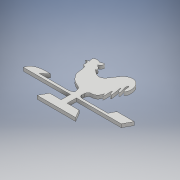
# Autodesk Inventor part: Part2
Saved by Autodesk Inventor 2017.1 (Build 211199000, 199)
## iProperties
Part Number: Part2
Material: 一般
Document SubType Name: Modeling
Designer: TomonoriSuzuki
Density: 1 g/cm^3
Appearance: 既定
Author: TomonoriSuzuki
Autodesk Inventor part; units mm, degrees
ref_plane "YZ Plane" through (0, 0, 0) normal (1, 0, 0) x (0, 1, 0)
ref_plane "XZ Plane" through (0, 0, 0) normal (0, 1, 0) x (-1, 0, 0)
ref_plane "XY Plane" through (0, 0, 0) normal (0, 0, 1) x (1, 0, 0)
sketch "スケッチ1" plane through (0, 0, 0) normal (0, 0, 1) x (1, 0, 0)
  line L0 (55.0072, -8.5794) -> (60.5037, 1.3591)
  line L1 (60.5037, 1.3591) -> (40.0223, 1.3591)
  line L2 (40.0223, 1.3591) -> (36.3075, -5.6978)
  line L3 (-44.8933, -5.4963) -> (-37.9032, 0.7038)
  line L4 (-37.9032, 0.7038) -> (-58.5109, 2.001) construction
  line L5 (-58.5109, 2.001) -> (-60.5622, -8.5794) construction
  spline S0 degree 2 poles (-37.9032, 0.7038) (-58.5109, 2.001) (-60.5622, -8.5794) knots 1 1 1 2 2 2
  line L6 (-15.656, 31.7874) -> (-2.1755, 18.5977) construction
  line L7 (-2.1755, 18.5977) -> (3.0159, 43.8698) construction
  line L8 (3.0159, 43.8698) -> (19.6839, 48.23) construction
  line L9 (19.6839, 48.23) -> (27.3182, 35.999) construction
  line L10 (27.3182, 35.999) -> (25.6769, 25.4506) construction
  line L11 (25.6769, 25.4506) -> (21.5058, 25.035) construction
  line L12 (21.5058, 25.035) -> (22.7873, 37.3838) construction
  line L13 (22.7873, 37.3838) -> (18.1485, 32.2406) construction
  line L14 (18.1485, 32.2406) -> (24.3226, 21.6179) construction
  line L15 (24.3226, 21.6179) -> (19.6839, 21.6179) construction
  line L16 (19.6839, 21.6179) -> (18.5132, 28.9494) construction
  line L17 (18.5132, 28.9494) -> (17.4163, 28.9494) construction
  line L18 (17.4163, 28.9494) -> (19.6839, 18.775) construction
  line L19 (19.6839, 18.775) -> (19.6839, 15.3221) construction
  spline S1 degree 4 poles (-15.656, 31.7874) (-2.1755, 18.5977) (3.0159, 43.8698) (19.6839, 48.23) (27.3182, 35.999) (25.6769, 25.4506) (21.5058, 25.035) (22.7873, 37.3838) (18.1485, 32.2406) (24.3226, 21.6179) (19.6839, 21.6179) (18.5132, 28.9494) (17.4163, 28.9494) (19.6839, 18.775) (19.6839, 15.3221) knots 1 1 1 1 1 2 3 4 5 6 7 8 9 10 11 12 12 12 12 12
  line L20 (19.6839, 15.3221) -> (18.1032, 13.7066) construction
  line L21 (18.1032, 13.7066) -> (16.92, 20.9253) construction
  line L22 (16.92, 20.9253) -> (15.2752, 20.6273) construction
  line L23 (15.2752, 20.6273) -> (16.92, 9.5318) construction
  line L24 (16.92, 9.5318) -> (15.3311, 6.9441) construction
  line L25 (15.3311, 6.9441) -> (14.2388, 16.1569) construction
  line L26 (14.2388, 16.1569) -> (14.2388, 5.6827) construction
  line L27 (14.2388, 5.6827) -> (6.7434, 3.9502) construction
  line L28 (6.7434, 3.9502) -> (3.9779, 5.6484) construction
  line L29 (3.9779, 5.6484) -> (2.3718, 1.2463) construction
  spline S2 degree 4 poles (19.6839, 15.3221) (18.1032, 13.7066) (16.92, 20.9253) (15.2752, 20.6273) (16.92, 9.5318) (15.3311, 6.9441) (14.2388, 16.1569) (14.2388, 5.6827) (6.7434, 3.9502) (3.9779, 5.6484) (2.3718, 1.2463) knots 1 1 1 1 1 2 3 4 5 6 7 8 8 8 8 8
  line L30 (2.3718, 1.2463) -> (2.0923, -2.1636) construction
  spline S3 degree 1 poles (2.3718, 1.2463) (2.0923, -2.1636) knots 1 1 2 2
  line L31 (-15.656, 31.7874) -> (-12.3988, 31.7874) construction
  line L32 (-12.3988, 31.7874) -> (-17.5466, 36.4877) construction
  line L33 (-17.5466, 36.4877) -> (-20.4147, 39.1064) construction
  line L34 (-20.4147, 39.1064) -> (-17.5466, 36.4877) construction
  line L35 (-17.5466, 36.4877) -> (-13.6458, 45.2036) construction
  line L36 (-13.6458, 45.2036) -> (-20.6141, 41.5266) construction
  line L37 (-20.6141, 41.5266) -> (-20.6142, 41.5266) construction
  line L38 (-20.6142, 41.5266) -> (-20.6136, 41.5266) construction
  line L39 (-20.6136, 41.5266) -> (-23.0367, 43.0844) construction
  line L40 (-23.0367, 43.0844) -> (-29.1871, 43.0844) construction
  line L41 (-29.1871, 43.0844) -> (-28.8447, 37.7285) construction
  line L42 (-28.8447, 37.7285) -> (-26.6696, 36.913) construction
  line L43 (-26.6696, 36.913) -> (-30.3539, 36.4706) construction
  line L44 (-30.3539, 36.4706) -> (-32.0674, 34.4706) construction
  line L45 (-32.0674, 34.4706) -> (-28.5043, 36.251) construction
  line L46 (-28.5043, 36.251) -> (-27.2474, 32.6902) construction
  line L47 (-27.2474, 32.6902) -> (-28.5043, 29.2574) construction
  line L48 (-28.5043, 29.2574) -> (-27.2474, 29.0008) construction
  line L49 (-27.2474, 29.0008) -> (-23.7709, 29.4706) construction
  line L50 (-23.7709, 29.4706) -> (-23.7709, 15.1294) construction
  line L51 (-23.7709, 15.1294) -> (-21.2036, 15.1294) construction
  line L52 (-21.2036, 15.1294) -> (-18.5996, 7.7294) construction
  line L53 (-18.5996, 7.7294) -> (-7.5699, 3.7053) construction
  line L54 (-7.5699, 3.7053) -> (-6.3253, 3.2512) construction
  line L55 (-6.3253, 3.2512) -> (-5.1075, -2.2999) construction
  spline S4 degree 4 poles (-15.656, 31.7874) (-12.3988, 31.7874) (-17.5466, 36.4877) (-20.4147, 39.1064) (-17.5466, 36.4877) (-13.6458, 45.2036) (-20.6141, 41.5266) (-20.6142, 41.5266) (-20.6136, 41.5266) (-23.0367, 43.0844) (-29.1871, 43.0844) (-28.8447, 37.7285) (-26.6696, 36.913) (-30.3539, 36.4706) (-32.0674, 34.4706) (-28.5043, 36.251) (-27.2474, 32.6902) (-28.5043, 29.2574) (-27.2474, 29.0008) (-23.7709, 29.4706) (-23.7709, 15.1294) (-21.2036, 15.1294) (-18.5996, 7.7294) (-7.5699, 3.7053) (-6.3253, 3.2512) (-5.1075, -2.2999) knots 1 1 1 1 1 2 3 4 5 6 7 8 9 10 11 12 13 14 15 16 17 18 19 20 21 22 23 23 23 23 23
  line L56 (-44.8933, -5.4963) -> (-13.2475, -5.4963)
  line L57 (36.3075, -5.6978) -> (6.9345, -5.6978)
  line L58 (6.9345, -5.6978) -> (2.0923, -5.6978) construction
  line L59 (2.0923, -5.6978) -> (2.0923, -2.1636) construction
  spline S5 degree 2 poles (6.9345, -5.6978) (2.0923, -5.6978) (2.0923, -2.1636) knots 1 1 1 2 2 2
  line L60 (-5.1075, -2.2999) -> (-5.1075, -5.4963) construction
  line L61 (-5.1075, -5.4963) -> (-13.2475, -5.4963) construction
  spline S6 degree 2 poles (-5.1075, -2.2999) (-5.1075, -5.4963) (-13.2475, -5.4963) knots 1 1 1 2 2 2
  line L62 (-60.5622, -8.5794) -> (-5.1075, -8.5794)
  line L63 (-5.1075, -8.5794) -> (-5.1075, -19.4842)
  line L64 (-5.1075, -19.4842) -> (-18.5996, -19.4842)
  line L65 (-18.5996, -19.4842) -> (-23.7709, -29.0905)
  line L66 (-23.7709, -29.0905) -> (21.621, -29.0905)
  line L67 (21.621, -29.0905) -> (16.0335, -19.4842)
  line L68 (16.0335, -19.4842) -> (2.0923, -19.4842)
  line L69 (2.0923, -19.4842) -> (2.0923, -8.5794)
  line L70 (2.0923, -8.5794) -> (55.0072, -8.5794)
  point P0 (0, 0)
  point P1 (0.2654, 30.4799)
  point P2 (3.1072, 34.6936)
  constraints: 30 end point, 9 horizontal, 6 vertical, 4 perpendicular, 4 point on line, 3 coincident, 1 parallel, 23 other
extrude "押し出し1" add sketch "スケッチ1" along normal blind 4
